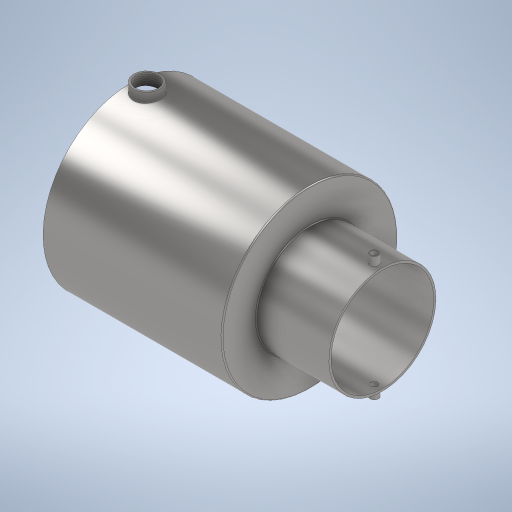
# Autodesk Inventor part: new outer wall
Saved by Autodesk Inventor 2023 (Build 270158000, 158)
## iProperties
Created: 2022-07-21
Part Number: new outer wall
Material: Stainless Steel
Document SubType Name: Modeling
Designer: station
Density: 8 g/cm^3
Appearance: Semi-Polished
Mass: 2032.08 g
Surface Area: 2551.28 cm^2
Volume: 254.01 cm^3
Author: station
Autodesk Inventor part; units mm, degrees
ref_plane "YZ Plane" through (0, 0, 0) normal (1, 0, 0) x (0, 1, 0)
sketch "Sketch1" plane through (0, 0, 0) normal (0, 0, 1) x (1, 0, 0)
  arc A0 (180.1312, 21.4516) -> (182.1847, 21.7676) centre (180.1312, 28.2803) ccw
  arc A1 (166.724, 25.044) -> (180.1312, 21.4516) centre (180.1312, 48.266) ccw
  line L0 (124.6541, 46.0566) -> (167.987, 21.0384)
  arc A2 (124.6541, 46.0566) -> (31.2848, 71.0749) centre (31.2848, -115.6637) ccw
  line L1 (1.263, 71.0749) -> (31.2848, 71.0749)
  line L2 (1.263, -0.4301) -> (1.263, 199.5699) construction
  line L3 (1.263, -0.4301) -> (320.4324, -0.4301)
  line L4 (1.263, 73.0749) -> (31.2848, 73.0749)
  arc A3 (125.6541, 47.7887) -> (31.2848, 73.0749) centre (31.2848, -115.6637) ccw
  line L5 (125.6541, 47.7887) -> (168.987, 22.7705)
  arc A4 (167.724, 26.7761) -> (180.1312, 23.4516) centre (180.1312, 48.266) ccw
  arc A5 (180.1312, 23.4516) -> (181.5842, 23.6753) centre (180.1312, 28.2803) ccw
  line L6 (182.1847, 21.7676) -> (237.115, 39.0871)
  line L7 (236.5136, 40.9945) -> (181.5833, 23.6751)
  arc A6 (180.1312, 23.4516) -> (181.5833, 23.6751) centre (180.1312, 28.2803) ccw
  line L8 (236.5136, 40.9945) -> (237.115, 39.0871)
  line L9 (1.263, 80.4749) -> (31.2848, 80.4749)
  line L10 (167.987, 21.0384) -> (167.987, -8.65)
  line L11 (31.2848, 80.4749) -> (166.987, 80.4749)
  line L12 (237.115, 39.0871) -> (234.2883, 48.052)
  line L13 (236.5136, 40.9945) -> (234.2883, 48.052)
  line L14 (234.2883, 48.052) -> (145.7323, 20.1304)
  line L15 (234.2883, 48.052) -> (238.3779, 48.052)
  line L16 (234.2883, 48.052) -> (168.987, 48.052)
  line L17 (168.987, 82.4749) -> (31.2848, 82.4749)
  line L18 (31.2848, 82.4749) -> (1.263, 82.4749)
  line L19 (234.2883, 50.052) -> (170.987, 50.052)
  line L20 (169.987, 21.0384) -> (169.987, 27.7779)
  line L21 (169.987, 51.052) -> (169.987, 81.4749)
  line L22 (167.987, 21.0384) -> (167.987, 27.1473)
  line L23 (167.987, 49.052) -> (167.987, 79.4749)
  arc A7 (167.987, 79.4749) -> (166.987, 80.4749) centre (166.987, 79.4749) ccw
  arc A8 (169.987, 81.4749) -> (168.987, 82.4749) centre (168.987, 81.4749) ccw
  arc A9 (169.987, 51.052) -> (170.987, 50.052) centre (170.987, 51.052) ccw
  arc A10 (167.987, 49.052) -> (168.987, 48.052) centre (168.987, 49.052) ccw
  line L24 (1.263, 80.4749) -> (1.263, 82.4749)
  line L25 (238.3779, 48.052) -> (238.3779, 50.052)
  line L26 (234.2883, 50.052) -> (238.3779, 50.052)
  line L27 (0, -0.4301) -> (371.9207, -0.4301)
  line L28 (0, 0) -> (5.3324, 0)
  dimension "d48" = 200
  dimension "d49" = 30.0219
  dimension "d50" = 186.7386
  dimension "d51" = 0
  dimension "d52" = 0
  dimension "d53" = 0
  dimension "d54" = 71.505
  dimension "d55" = 2
  dimension "d56" = 2
  dimension "d57" = 2
  dimension "d58" = 2
  dimension "d59" = 2
  dimension "d60" = 17.5
  dimension "d61" = 54.9303
  dimension "d62" = 2
  dimension "d63" = 7.4
  dimension "d66" = 7.4
  dimension "d67" = 17.5
  dimension "d68" = 2
  dimension "d69" = 2
  dimension "d70" = 1
  dimension "d71" = 1
  dimension "d72" = 1
  dimension "d73" = 1
  dimension "d158" = 0.4301
  dimension "d160" = 50.052
  constraints: 58 end point, 22 point on circle, 11 centre point, 9 tangent, 5 horizontal, 4 parallel, 4 vertical, 3 point on line, 1 collinear, 1 perpendicular, 2 other
  measures "d48" distance of L2.start L2.end
  measures "d49" distance of L1.start L1.end
  measures "d50" radius of A2
  measures "d51" distance from line of L1.start L2
  measures "d52" distance of A2.end L1.end
  measures "d53" distance of L0.start A2.start
  measures "d54" distance between parallel lines of L3 L1
  measures "d55" distance between parallel lines of L1 L4
  measures "d56" radial gap between concentric circles of A2 A3
  measures "d57" distance between parallel lines of L0 L5
  measures "d58" radial gap between concentric circles of A1 A4
  measures "d59" radial gap between concentric circles of A0 A5
  measures "d60" angle of L3 L6
  measures "d61" horizontal distance of L6.start L6.end
  measures "d62" distance between parallel lines of L6 L7
  measures "d63" distance between parallel lines of L4 L9
  measures "d66" distance of L12.end L7.start
  measures "d67" angle of L3 L14
  measures "d68" distance between parallel lines of L11 L17
  measures "d69" distance between parallel lines of L16 L19
  measures "d70" radius of A7
  measures "d71" radius of A8
  measures "d72" radius of A9
  measures "d73" radius of A10
  measures "d158" distance between parallel lines of L3 L28
  measures "d160" distance between parallel lines of L28 L26
revolve "Revolution3" add sketch "Sketch1" angle 360 about axis through (1.263, -0.4301, 0) along (1, 0, 0) contours L16 A10 L23 A7 L11 L9 L24 L18 L17 A8 L21 A9 L19 L26 L25 L15
sketch "Sketch5" plane through (0, 0, 0) normal (0, 0, 1) x (1, 0, 0)
  point P0 (0, 0)
ref_plane "Work Plane6" through (0, 82.905, 0) normal (0, 1, 0) x (-1, 0, 0)
sketch "Sketch12" plane through (0, 82.905, 0) normal (0, 1, 0) x (-1, 0, 0)
  line L0 (0, 0) -> (-1.263, 0)
  line L1 (-1.263, 82.905) -> (-1.263, -82.905) projected
  line L2 (-1.263, 0) -> (-31.263, 0) construction
  line L3 (-31.263, 0) -> (-16.263, 0) construction
  circle A0 centre (-16.263, 0) radius 12.5
  circle A1 centre (-16.263, 0) radius 10.668
  dimension "d141" = 30
  dimension "d142" = 15
  dimension "d143" = 25
  dimension "d144" = 21.336
  constraints: 6 end point, 2 centre point, 2 coincident, 2 midpoint, 1 point on line
  measures "d141" distance of L0.end L2.end
  measures "d142" distance of L2.end L3.end
  measures "d143" diameter of A0
  measures "d144" diameter of A1
extrude "Extrusion6" add sketch "Sketch12" along normal blind 8 and the other way blind 2
extrude "Extrusion7" cut sketch "Sketch12" against normal blind 168 contours A1
thread "Thread11" size "M22x1.5" class "6H" standard "ANSI Metric M Profile" full length
pattern_circular "Circular Pattern1" count 2 over 360 about axis through (-10, 0, 0) along (1, 0, 0) of "Extrusion6"
thread "Thread12" size "M22x1.5" class "6H" standard "ANSI Metric M Profile" full length
ref_plane "Work Plane7" through (0, 50.052, 0) normal (0, 1, 0) x (-1, 0, 0)
sketch "Sketch13" plane through (0, 50.052, 0) normal (0, 1, 0) x (-1, 0, 0)
  line L0 (-238.3779, 50.4822) -> (-238.3779, -50.4822) projected
  line L1 (-238.3779, 0) -> (-230.7769, 0) construction
  circle A0 centre (-230.7769, 0) radius 3
  circle A1 centre (-230.7769, 0) radius 4
  point P0 (0, 0)
  dimension "d161" = 7.601
  dimension "d162" = 6
  dimension "d163" = 8
  constraints: 2 centre point, 2 coincident, 2 end point, 1 horizontal, 1 midpoint
  measures "d161" distance of L1.start L1.end
  measures "d162" diameter of A0
  measures "d163" diameter of A1
extrude "Extrusion8" add sketch "Sketch13" along normal blind 8 and the other way blind 2
pattern_circular "Circular Pattern2" count 2 over 360 about axis through (203.6824, -0.4301, 0) along (1, 0, 0) of "Extrusion8"
extrude "Extrusion9" cut sketch "Sketch13" along normal blind 10 and the other way blind 145 contours A0
thread "Thread13" size "M6x1" class "6H" standard "ANSI Metric M Profile" full length
thread "Thread14" size "M6x1" class "6H" standard "ANSI Metric M Profile" full length
body "Solid3"
